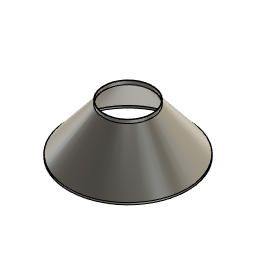
2023_05_24_AirFlowCylinder v2 (Autodesk Fusion 360 design; units mm, degrees)
Autodesk Fusion 360 part; units mm, degrees
sketch "Sketch1" plane through (0, 0, 0) normal (0, 0, 1) x (1, 0, 0)
  circle A0 centre (0, 0) radius 95
  circle A1 centre (0, 0) radius 97.5
  dimension "d1" = 190
  dimension "d2" = 195
  constraint coincident A0.centre A1.centre
  measures "d1" diameter of A0
  measures "d2" diameter of A1
extrude "Extrude1" add sketch "Sketch1" along normal blind 3 makes body 1
sketch "Sketch2" plane through (0, 0, 0) normal (0, 0, 1) x (1, 0, 0)
  circle A0 centre (0, 0) radius 37.5
  circle A1 centre (0, 0) radius 39
  dimension "d5" = 75
  dimension "d6" = 78
  constraint coincident A0.centre A1.centre
  constraint concentric A0 A1
  measures "d5" diameter of A0
  measures "d6" diameter of A1
extrude "Extrude2" add sketch "Sketch2" along normal blind 20 separate body makes body 2
move_body "Move1" bodies 2 to x (1, 0, 0) y (0, 1, 0) z (0, 0, 1) at (0, 0, 40)
sketch "Sketch3" plane through (0, 0, 0) normal (0, 1, 0) x (1, 0, 0)
  line L0 (0, 0) -> (-97.7336, 0)
  line L1 (-97.7336, 0) -> (-97.7336, -3.0833)
  line L2 (-97.7336, -3.0833) -> (-39.9169, -74.481)
  line L3 (-39.9169, -74.481) -> (-39.9169, -80)
  line L4 (-39.9169, -80) -> (-39, -80)
  line L5 (-39, -80) -> (-39, -74)
  line L6 (-39, -74) -> (-96.816, -3.0833)
  line L7 (-96.816, -3.0833) -> (-96.816, 0)
  line L8 (-97.7336, 0) -> (-96.816, 0)
  dimension "d9" = 141
  constraint coincident L0.start origin
  constraint horizontal L0
  constraint perpendicular L0 L1
  constraint perpendicular L0 L3
  constraint perpendicular L3 L4
  constraint perpendicular L4 L5
  constraint coincident L0 L7.end
  constraint perpendicular L0 L7
  measures "d9" angle of L1 L2
revolve "Revolve1" add sketch "Sketch3" angle 360 about axis through (0, 0, 1.75) along (0, 0, 1) separate body makes body 3
sketch "Sketch4" plane through (0, 0, 0) normal (0, 0, 1) x (1, 0, 0)
hidden bodies 1 2
equation "d9 = 90 deg + 51 deg"
